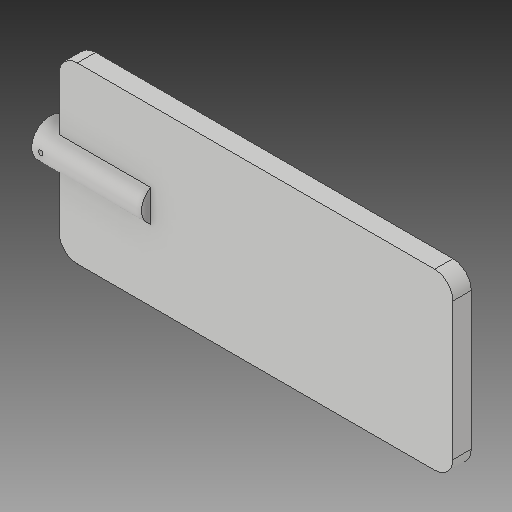
# Autodesk Inventor part: UntererRührer
Saved by Autodesk Inventor 2017 (Build 210142000, 142)
## iProperties
Created: 2019-06-21
Part Number: UntererRührer
Material: Generic
Document SubType Name: Modeling
Designer: Ole Simmering
Density: 1 g/cm^3
Appearance: Default
Author: Ole Simmering
Autodesk Inventor part; units mm, degrees
ref_plane "YZ Plane" through (0, 0, 0) normal (1, 0, 0) x (0, 1, 0)
ref_plane "XZ Plane" through (0, 0, 0) normal (0, 1, 0) x (-1, 0, 0)
sketch "Sketch1" plane through (0, 0, 0) normal (0, 0, 1) x (1, 0, 0)
  line L0 (0, 0) -> (43, 0)
  line L1 (43, 0) -> (43, 19)
  line L2 (43, 19) -> (0, 19)
  line L3 (0, 19) -> (0, 0)
  dimension "d0" = 43
  constraints: 8 end point, 2 parallel, 1 horizontal, 1 perpendicular
  measures "d0" distance of L0.start L0.end
extrude "Extrusion1" add sketch "Sketch1" along normal blind 2
fillet "Fillet1" radius 2 4 edges at (43, 19, 1) (43, 0, 1) (0, 19, 1) (0, 0, 1)
sketch "Sketch3" plane through (0, 2, 0) normal (-1, 0, 0) x (0, 0, 1)
  line L0 (2, 0) -> (0, 0) construction
  line L1 (2, 15) -> (2, 0) construction
  line L2 (0, 0) -> (2, 15) construction
  line L3 (0, 15) -> (2, 0) construction
  circle A0 centre (1, 7.5) radius 2
  point P0 (0, -2)
  dimension "d4" = 4
  constraints: 4 end point, 1 centre point, 1 midpoint
  measures "d4" diameter of A0
extrude "Extrusion2" add sketch "Sketch3" along normal blind 2 and the other way blind 10
sketch "Sketch4" plane through (-2, 9.5, 1) normal (-1, 0, 0) x (0, 0, 1)
  point P0 (-1, -9.5)
  point P1 (0, 0)
hole "Hole1" at (-2, 9.5, 1) direction (1, 0, 0) diameter 2.85 depth 10.4 tip angle 118 thread size "M3.5x0.6" class "6H" standard "ANSI Metric M Profile"
ref_plane "Work Plane2" through (0, 0, 3) normal (0, 0, 1) x (1, 0, 0)
ref_plane "Work Plane1" through (0, 0, 1) normal (0, 0, 1) x (1, 0, 0)
sketch "Sketch6" plane through (0, 0, 3) normal (0, 0, 1) x (1, 0, 0)
  line L0 (-2, 11.5) -> (-2, 7.5) construction
  line L1 (0, 7.5) -> (0, 7.7679) construction
  line L2 (-2, 11.5) -> (0, 7.5) construction
  line L3 (0, 7.5) -> (-2, 7.5) construction
  line L4 (-2, 7.5) -> (0, 11.5) construction
  line L5 (0, 11.5) -> (-2, 11.5) construction
  point P0 (0, 0)
  point P1 (-1, 9.5)
  constraints: 6 end point, 1 midpoint, 1 perpendicular, 1 point on line
hole "Hole2" at (-1, 9.5, 3) direction (0, 0, -1) diameter 0.5 depth 3.5 tip angle 118
body "Solid1"
